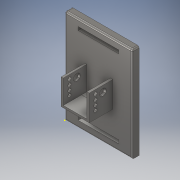
# Autodesk Inventor part: LucasCharles Part 1 wall mount FINAL v2
Saved by Autodesk Inventor 2018 (Build 220112000, 112)
## iProperties
Created: 2018-05-14
Part Number: LucasCharles Part 1 wall mount FINAL v2
Material: Stainless Steel, Austenitic
Document SubType Name: Modeling
Designer: 21lsilva
Density: 8 g/cm^3
Appearance: Semi-Polished
Author: 21lsilva
Autodesk Inventor part; units mm, degrees
ref_plane "YZ Plane" through (0, 0, 0) normal (1, 0, 0) x (0, 1, 0)
ref_plane "XZ Plane" through (0, 0, 0) normal (0, 1, 0) x (-1, 0, 0)
ref_plane "XY Plane" through (0, 0, 0) normal (0, 0, 1) x (1, 0, 0)
sketch "Sketch1" plane through (0, 0, 0) normal (0, 0, 1) x (1, 0, 0)
  line L0 (0, 0) -> (127, 0)
  line L1 (127, 0) -> (127, 177.8)
  line L2 (127, 177.8) -> (0, 177.8)
  line L3 (0, 177.8) -> (0, 0)
  dimension "d0" = 127
  dimension "d1" = 177.8
  constraints: 8 end point, 2 parallel, 1 horizontal, 1 perpendicular
  measures "d0" distance of L2.end L1.end
  measures "d1" distance of L1.end L0.end
extrude "Extrusion1" add sketch "Sketch1" against normal blind 12.7
sketch "Sketch2" plane through (0, 0, 0) normal (0, 0, 1) x (1, 0, 0)
  line L0 (0, 0) -> (0, 177.8) projected
  line L1 (127, 177.8) -> (127, 0) projected
  line L2 (25.4, 158.75) -> (101.6, 158.75)
  line L3 (101.6, 158.75) -> (101.6, 165.1)
  line L4 (101.6, 165.1) -> (25.4, 165.1)
  line L5 (25.4, 165.1) -> (25.4, 158.75)
  line L6 (25.4, 19.05) -> (101.6, 19.05)
  line L7 (101.6, 19.05) -> (101.6, 12.7)
  line L8 (101.6, 12.7) -> (25.4, 12.7)
  line L9 (25.4, 12.7) -> (25.4, 19.05)
  point P0 (63.5, 158.75)
  point P1 (101.6, 158.75)
  point P2 (63.5, 41.3327)
  dimension "d25" = 6.35
  dimension "d26" = 6.35
  constraints: 16 end point, 4 parallel, 2 horizontal, 2 perpendicular
  measures "d25" distance of L3.end L2.end
  measures "d26" distance of L6.end L7.end
sketch "Sketch3" plane through (0, 0, 0) normal (0, 0, 1) x (1, 0, 0)
  point P0 (0, 0)
sketch "Sketch4" plane through (0, 0, 0) normal (0, 0, 1) x (1, 0, 0)
  line L0 (38.1, 63.5) -> (90.6923, 63.5)
  line L1 (90.6923, 63.5) -> (90.6923, 111.7968)
  line L2 (90.6923, 111.7968) -> (38.1, 111.7968)
  line L3 (38.1, 111.7968) -> (38.1, 63.5)
  point P0 (0, 0)
  constraints: 8 end point, 2 parallel, 1 horizontal, 1 perpendicular
extrude "Extrusion2" add sketch "Sketch4" along normal blind 44.45
sketch "Sketch5" plane through (38.1, 63.5, 0) normal (-1, 0, 0) x (0, 0, 1)
  circle A0 centre (19.05, 37.0546) radius 6.35
  circle A1 centre (33.02, 41.2603) radius 3.175
  circle A2 centre (33.02, 31.5839) radius 3.175
  circle A3 centre (33.02, 23.1169) radius 3.175
  circle A4 centre (33.02, 14.4772) radius 3.175
  circle A5 centre (33.02, 5.8375) radius 3.175
  line L0 (0, 114.3) -> (0, -63.5) projected
  line L1 (44.45, 48.2968) -> (44.45, 0) projected
  dimension "d10" = 6.35
  dimension "d29" = 19.05
  dimension "d30" = 11.43
  dimension "d31" = 11.43
  dimension "d32" = 11.43
  dimension "d33" = 11.43
  dimension "d34" = 11.43
  constraints: 6 centre point, 5 coincident
  measures "d10" diameter of A1
  measures "d29" distance from line of L0 A0.centre
  measures "d30" distance from line of L1 point (33.02, 41.26)
  measures "d31" distance from line of L1 A2.centre
  measures "d32" distance from line of L1 A3.centre
  measures "d33" distance from line of L1 A4.centre
  measures "d34" distance from line of L1 point (33.02, 5.838)
extrude "Extrusion3" cut sketch "Sketch5" against normal blind 254 contours A0
extrude "Extrusion5" cut sketch "Sketch5" against normal blind 254 contours A1 | A2 | A3 | A4
sketch "Sketch6" plane through (0, 0, 44.45) normal (0, 0, 1) x (1, 0, 0)
  line L0 (38.1, 107.9353) -> (90.6923, 107.9353) projected
  line L1 (41.91, 67.31) -> (86.0576, 67.31)
  line L2 (86.0576, 67.31) -> (86.0576, 107.9353)
  line L3 (86.0576, 107.9353) -> (41.91, 107.9353)
  line L4 (41.91, 107.9353) -> (41.91, 67.31)
  point P0 (0, 0)
  constraints: 8 end point, 2 parallel, 1 horizontal, 1 perpendicular, 1 point on line
extrude "Extrusion6" cut sketch "Sketch6" against normal blind 34.29
sketch "Sketch7" plane through (38.1, 111.7968, 0) normal (0, 1, 0) x (1, 0, 0)
  line L0 (3.81, -44.45) -> (3.81, -33.02) projected
  line L1 (3.81, -10.16) -> (47.9576, -10.16) projected
  line L2 (3.81, -38.735) -> (47.9576, -38.735)
  line L3 (47.9576, -38.735) -> (47.9576, -10.16)
  line L4 (47.9576, -10.16) -> (3.81, -10.16)
  line L5 (3.81, -10.16) -> (3.81, -38.735)
  line L6 (3.81, -38.735) -> (47.9576, -38.735)
  line L7 (47.9576, -38.735) -> (47.9576, -50.1618)
  line L8 (47.9576, -50.1618) -> (3.81, -50.1618)
  line L9 (3.81, -50.1618) -> (3.81, -38.735)
  point P0 (-38.1, 0)
  constraints: 16 end point, 4 parallel, 2 horizontal, 2 perpendicular, 1 midpoint
extrude "Extrusion7" cut sketch "Sketch7" against normal blind 34.29 contours L0 L5 L1 L3 L2
extrude "Extrusion8" cut sketch "Sketch7" against normal blind 34.29 contours L0 L2 L7 L8 L9
extrude "Extrusion11" cut sketch "Sketch2" against normal blind 25.4
sketch "Sketch8" plane through (38.1, 111.7968, 0) normal (0, 1, 0) x (1, 0, 0)
  line L0 (47.9576, -10.16) -> (3.81, -10.16) projected
  line L1 (63.5, 0) -> (-12.7, 0) projected
  line L2 (3.81, -10.16) -> (47.9681, -10.16)
  line L3 (47.9681, -10.16) -> (47.9681, 0)
  line L4 (47.9681, 0) -> (3.81, 0)
  line L5 (3.81, 0) -> (3.81, -10.16)
  point P0 (-38.1, 0)
  constraints: 8 end point, 2 parallel, 1 horizontal, 1 perpendicular, 1 point on line
extrude "Extrusion12" cut sketch "Sketch8" against normal blind 44.45
fillet "Fillet1" radius 3.175 6 edges at (0, 177.8, -6.35) (127, 177.8, -6.35) (63.5, 177.8, 0) (127, 88.9, 0) (0, 88.9, 0) (63.5, 0, 0)
body "Solid1"
